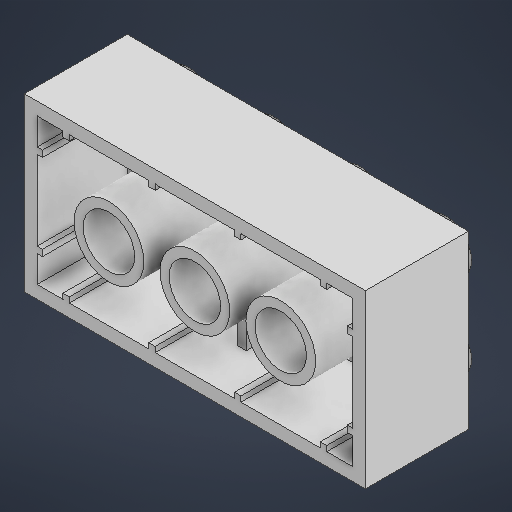
# Autodesk Inventor part: Lego
Saved by Autodesk Inventor 2025.4 (Build 294407000, 407)
## iProperties
Created: 2026-05-15
Part Number: Lego
Material: Generic
Document SubType Name: Modeling
Designer: VuQuan
Density: 1 g/cm^3
Appearance: Default
Author: VuQuan
Autodesk Inventor part; units mm, degrees
ref_plane "YZ Plane" through (0, 0, 0) normal (1, 0, 0) x (0, 1, 0)
ref_plane "XZ Plane" through (0, 0, 0) normal (0, 1, 0) x (-1, 0, 0)
ref_plane "XY Plane" through (0, 0, 0) normal (0, 0, 1) x (1, 0, 0)
sketch "Sketch1" plane through (0, 0, 0) normal (0, 0, 1) x (1, 0, 0)
  line L0 (0, 0) -> (31.8, 0)
  line L1 (31.8, 0) -> (31.8, 16)
  line L2 (31.8, 16) -> (0, 16)
  line L3 (0, 16) -> (0, 0)
  circle A0 centre (3.9, 4) radius 2.4
  circle A1 centre (11.9, 4) radius 2.4
  circle A2 centre (19.9, 4) radius 2.4
  circle A3 centre (27.9, 4) radius 2.4
  circle A4 centre (3.9, 12) radius 2.4
  circle A5 centre (11.9, 12) radius 2.4
  circle A6 centre (19.9, 12) radius 2.4
  circle A7 centre (27.9, 12) radius 2.4
  dimension "d0" = 31.8
  dimension "d1" = 16
  dimension "d2" = 4.8
  dimension "d3" = 4
  dimension "d4" = 3.9
  dimension "d7" = 8
  dimension "d10" = 8
  constraints: 8 centre point, 8 end point, 2 horizontal, 2 parallel, 1 perpendicular, 1 vertical, 14 other
  measures "d0" distance of L2.end L1.end
  measures "d1" distance of L1.end L0.end
  measures "d2" diameter of A0
  measures "d3" distance from line of L0 A0.centre
  measures "d4" distance from line of A0.centre L3
  measures "d7" distance of A0.centre A1.centre
  measures "d10" distance of A0.centre A4.centre
extrude "Extrusion1" add sketch "Sketch1" along normal blind 9.6 contours L3 L2 L1 L0 | A0 | A1 | A2 | A3 | A4 | A5 | A6 | A7
extrude "Extrusion2" add sketch "Sketch1" against normal blind 1.8 contours A0 | A1 | A2 | A3 | A4 | A5 | A6 | A7
sketch "Sketch2" plane through (0, 0, 9.6) normal (0, 0, 1) x (1, 0, 0)
  line L0 (31.8, 0) -> (31.8, 16) projected
  line L1 (31.8, 16) -> (0, 16) projected
  line L2 (0, 16) -> (0, 0) projected
  line L3 (0, 0) -> (31.8, 0) projected
  line L4 (30.6, 1.2) -> (30.6, 14.8)
  line L5 (30.6, 14.8) -> (1.2, 14.8)
  line L6 (1.2, 14.8) -> (1.2, 1.2)
  line L7 (1.2, 1.2) -> (30.6, 1.2)
  line L8 (28.2, 1.2) -> (28.2, 1.7)
  line L9 (28.2, 1.7) -> (27.6, 1.7)
  line L10 (27.6, 1.7) -> (27.6, 1.2)
  circle A0 centre (27.9, 4) radius 2.4 projected
  line L11 (30.6, 3.7) -> (30.1, 3.7)
  line L12 (30.1, 3.7) -> (30.1, 4.3)
  line L13 (30.1, 4.3) -> (30.6, 4.3)
  circle A1 centre (19.9, 4) radius 2.4 projected
  line L14 (20.2, 1.2) -> (20.2, 1.7)
  line L15 (20.2, 1.7) -> (19.6, 1.7)
  line L16 (19.6, 1.7) -> (19.6, 1.2)
  line L17 (15.9, 1.2) -> (15.9, 14.8) construction
  line L18 (1.2, 8) -> (15.9, 8) construction
  line L19 (3.6, 1.2) -> (3.6, 1.7)
  line L20 (3.6, 1.7) -> (4.2, 1.7)
  line L21 (4.2, 1.7) -> (4.2, 1.2)
  line L22 (1.2, 3.7) -> (1.7, 3.7)
  line L23 (1.7, 3.7) -> (1.7, 4.3)
  line L24 (1.7, 4.3) -> (1.2, 4.3)
  line L25 (11.6, 1.2) -> (11.6, 1.7)
  line L26 (11.6, 1.7) -> (12.2, 1.7)
  line L27 (12.2, 1.7) -> (12.2, 1.2)
  line L28 (28.2, 14.8) -> (28.2, 14.3)
  line L29 (28.2, 14.3) -> (27.6, 14.3)
  line L30 (27.6, 14.3) -> (27.6, 14.8)
  line L31 (30.6, 12.3) -> (30.1, 12.3)
  line L32 (30.1, 12.3) -> (30.1, 11.7)
  line L33 (30.1, 11.7) -> (30.6, 11.7)
  line L34 (20.2, 14.8) -> (20.2, 14.3)
  line L35 (20.2, 14.3) -> (19.6, 14.3)
  line L36 (19.6, 14.3) -> (19.6, 14.8)
  line L37 (12.2, 14.3) -> (12.2, 14.8)
  line L38 (11.6, 14.3) -> (12.2, 14.3)
  line L39 (11.6, 14.8) -> (11.6, 14.3)
  line L40 (4.2, 14.3) -> (4.2, 14.8)
  line L41 (3.6, 14.3) -> (4.2, 14.3)
  line L42 (3.6, 14.8) -> (3.6, 14.3)
  line L43 (1.7, 12.3) -> (1.7, 11.7)
  line L44 (1.7, 11.7) -> (1.2, 11.7)
  line L45 (1.2, 12.3) -> (1.7, 12.3)
  circle A2 centre (15.9, 8) radius 2.4
  circle A3 centre (15.9, 8) radius 3.25
  line L46 (15.9, 8) -> (30.6, 8) construction
  circle A4 centre (23.9097, 8) radius 2.4
  circle A5 centre (23.9097, 8) radius 3.25
  circle A6 centre (7.8903, 8) radius 2.4
  circle A7 centre (7.8903, 8) radius 3.25
  line L47 (15.5, 1.2) -> (15.5, 4.7747)
  line L48 (16.3, 1.2) -> (16.3, 4.7747)
  line L49 (15.5, 11.2253) -> (15.5, 14.8)
  line L50 (16.3, 11.2253) -> (16.3, 14.8)
  point P0 (27.9, 1.7)
  point P1 (30.1, 4)
  point P2 (19.9, 1.7)
  point P3 (3.9, 1.7)
  point P4 (1.7, 4)
  point P5 (11.9, 1.7)
  point P6 (27.9, 14.3)
  point P7 (30.1, 12)
  point P8 (19.9, 14.3)
  point P9 (11.9, 14.3)
  point P10 (3.9, 14.3)
  point P11 (1.7, 12)
  dimension "d18" = 1.2
  dimension "d19" = 0.6
  dimension "d20" = 0.5
  dimension "d21" = 4.8
  dimension "d22" = 6.5
  dimension "d23" = 0.8
  constraints: 92 end point, 47 symmetric about line, 8 midpoint, 6 centre point, 6 equal length, 6 vertical, 5 perpendicular, 5 point on line, 4 point on circle, 3 coincident, 2 collinear, 2 equal radius, 2 vertical alignment, 1 horizontal, 1 horizontal alignment, 1 parallel, 1 tangent, 15 other
  measures "d19" distance between parallel lines of L10 L8
  measures "d21" diameter of A2
  measures "d22" diameter of A3
  measures "d23" distance between parallel lines of L47 L48
extrude "Extrusion3" cut sketch "Sketch2" against normal blind 8.4 contours L7 L8 A0 L11 L4 | L13 A0 L10 L7 L14 A1 L16 L48 A3 L50 L5 L36 L35 L34 L30 L29 L28 L4 L31 L32 L33 | A0 L8 L9 L10 L13 L12 L11 | L14 L15 L16 A1 | L7 L27 L26 L25 L21 L20 L19 L6 L22 L23 L24 L44 L43 L45 L5 L42 L41 L40 L39 L38 L37 L49 A3 L47 | A2 | A4 | A6 picked at (19.8049, 3.261)
extrude "Extrusion4" cut sketch "Sketch2" against normal blind 4.4 contours L7 L47 A3 L48 | L49 L5 L50 A3
shell "Shell2" thickness 1.4 removed faces 2 at (23.7727, 13.6088, 1.2) at (8.0273, 13.6088, 1.2)
body "Solid1"
